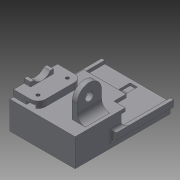
# Autodesk Inventor part: MotorHolder
Saved by Autodesk Inventor 2013 (Build 170138000, 138)
## iProperties
Created: 2013-11-09
Part Number: MotorHolder
Material: Generic
Document SubType Name: Modeling
Designer: JustinIndra
Density: 1 g/cm^3
Author: JustinIndra
Autodesk Inventor part; units mm, degrees
ref_plane "YZ Plane" through (0, 0, 0) normal (1, 0, 0) x (0, 1, 0)
ref_plane "XZ Plane" through (0, 0, 0) normal (0, 1, 0) x (-1, 0, 0)
ref_plane "XY Plane" through (0, 0, 0) normal (0, 0, 1) x (1, 0, 0)
sketch "Sketch1" plane through (0, 0, 0) normal (0, 1, 0) x (-1, 0, 0)
  line L0 (20, 0) -> (-20, 0)
  line L1 (-20, 0) -> (-20, 10)
  line L2 (-20, 10) -> (20, 10)
  line L3 (20, 10) -> (20, 0)
  circle A0 centre (0, 0) radius 3.175
  arc A1 (-20, 0) -> (20, 0) centre (0, 16.3026) ccw
  line L4 (20, 0) -> (-20, 0)
  line L5 (13.2784, -9.5) -> (-17.2645, -9.5) construction
  line L6 (20, 10) -> (-20, 10)
  line L7 (-20, 10) -> (-20, -10)
  line L8 (-20, -10) -> (20, -10)
  line L9 (20, -10) -> (20, 10)
  dimension "d0" = 40
  dimension "d2" = 6.35
  dimension "d4" = 9.5
  dimension "d5" = 10
  dimension "d6" = 20
  constraints: 20 end point, 5 parallel, 3 coincident, 3 perpendicular, 2 centre point, 2 horizontal, 2 point on circle, 1 collinear, 1 midpoint, 1 tangent
  measures "d0" distance of L1.end L2.end
  measures "d2" diameter of A0
  measures "d4" distance between parallel lines of L5 L0
  measures "d5" distance of L0.end L1.end
  measures "d6" distance of L8.end L2.end
extrude "Extrusion1" add sketch "Sketch1" along normal mid plane 8.5 contours L9 L8 L7 A1
sketch "Sketch2" plane through (0, -4.25, 0) normal (0, -1, 0) x (1, 0, 0)
  line L0 (20, -10) -> (20, 0) projected
  line L1 (-20, -10) -> (20, -10)
  line L2 (20, -10) -> (20, 10)
  line L3 (20, 10) -> (-20, 10)
  line L4 (-20, 10) -> (-20, -10)
  point P0 (0, 0)
  dimension "d9" = 20
  constraints: 8 end point, 2 parallel, 1 collinear, 1 horizontal, 1 perpendicular
  measures "d9" distance of L3.end L1.start
extrude "Extrusion2" add sketch "Sketch2" along normal blind 2
sketch "Sketch4" plane through (0, -4.25, 0) normal (0, 1, 0) x (1, 0, 0)
  circle A0 centre (0, 0) radius 3.175
  dimension "d12" = 6.35
  constraints: 1 centre point, 1 coincident
  measures "d12" diameter of A0
extrude "Extrusion3" cut sketch "Sketch4" against normal through all
mirror "Mirror1" about plane through (0, 0, 0) normal (0, 1, 0) of "Extrusion2", "Extrusion3"
sketch "Sketch5" plane through (0, -6.25, 0) normal (0, -1, 0) x (1, 0, 0)
  line L0 (-20, -10) -> (20, -10) projected
  line L1 (-20, 10) -> (-13, 10)
  line L2 (-13, 10) -> (-13, 2.5)
  line L3 (-13, 2.5) -> (-20, 2.5)
  line L4 (-20, 2.5) -> (-20, 10)
  dimension "d15" = 7
  dimension "d17" = 12.5
  constraints: 8 end point, 2 parallel, 1 horizontal, 1 perpendicular
  measures "d15" distance of L2.end L3.end
  measures "d17" distance between parallel lines of L3 L0
extrude "Extrusion4" cut sketch "Sketch5" against normal up to next
mirror "Mirror2" about plane through (0, 0, 0) normal (1, 0, 0) of "Extrusion4"
sketch "Sketch6" plane through (20, -6.25, -10) normal (0, 0, -1) x (-1, 0, 0)
  line L0 (40, 0) -> (40, 12.5) projected
  line L1 (0, 0) -> (40, 0)
  line L2 (40, 0) -> (40, 12.5)
  line L3 (40, 12.5) -> (0, 12.5)
  line L4 (0, 12.5) -> (0, 0)
  point P0 (20, 6.25)
  dimension "d20" = 12.5
  constraints: 8 end point, 2 parallel, 1 horizontal, 1 perpendicular, 1 point on line
  measures "d20" distance of L3.end L1.start
extrude "Extrusion5" add sketch "Sketch6" along normal blind 18.25
sketch "Sketch7" plane through (0, -6.25, 0) normal (0, -1, 0) x (1, 0, 0)
  circle A0 centre (0, 0) radius 3.175 projected
  line L0 (-7.5, -5) -> (-4.5, -5)
  line L1 (-4.5, -5) -> (-4.5, -20)
  line L2 (-4.5, -20) -> (-7.5, -20)
  line L3 (-7.5, -20) -> (-7.5, -5)
  line L4 (10, -5) -> (13, -5)
  line L5 (13, -5) -> (13, -20)
  line L6 (13, -20) -> (10, -20)
  line L7 (10, -20) -> (10, -5)
  dimension "d23" = 15
  dimension "d25" = 3
  dimension "d26" = 4.5
  dimension "d27" = 5
  dimension "d28" = 14.5
  constraints: 16 end point, 4 parallel, 2 equal length, 2 horizontal, 2 perpendicular, 1 collinear
  measures "d23" distance of L2.end L0.start
  measures "d25" distance of L1.end L2.end
  measures "d26" distance from line of A0.centre L1
  measures "d27" distance from line of A0.centre L0
  measures "d28" distance between parallel lines of L1 L7
extrude "Extrusion6" add sketch "Sketch7" along normal blind 17.5 contours L4 L5 L6 L7
sketch "Sketch8" plane through (10, -6.25, -20) normal (-1, 0, 0) x (0, 0, 1)
  line L0 (15, -17.5) -> (0, -17.5)
  circle A0 centre (7.5, -10) radius 2.55
  line L1 (0, 0) -> (15, 0) projected
  line L2 (0, 0) -> (0, -17.5) projected
  line L3 (15, -17.5) -> (0, -17.5) projected
  line L4 (15, 0) -> (15, -17.5) projected
  point P0 (20, 6.25)
  point P1 (7.5, -17.5)
  dimension "d31" = 5.1
  dimension "d34" = 7.5
  constraints: 2 end point, 1 centre point, 1 midpoint, 1 vertical alignment
  measures "d31" diameter of A0
  measures "d34" distance from line of L0 A0.centre
extrude "Extrusion7" cut sketch "Sketch8" against normal through all contours A0
fillet "Fillet1" radius 7.5 2 edges at (11.5, -23.75, -5) (11.5, -23.75, -20)
sketch "Sketch9" plane through (0, -6.25, 0) normal (0, -1, 0) x (1, 0, 0)
  line L0 (10, -20) -> (10, -5) projected
  line L1 (-20, 1) -> (-5, 1)
  line L2 (-5, 1) -> (-5, -26)
  line L3 (-5, -26) -> (-20, -26)
  line L4 (-20, -26) -> (-20, 1)
  line L5 (-20, 2.5) -> (-20, -28.25) projected
  point P0 (-5, -12.5)
  point P1 (10, -12.5)
  dimension "d38" = 15
  dimension "d39" = 27
  constraints: 8 end point, 2 midpoint, 2 parallel, 1 collinear, 1 horizontal, 1 horizontal alignment, 1 perpendicular
  measures "d38" distance between parallel lines of L0 L2
  measures "d39" distance of L3.end L1.start
extrude "Extrusion8" add sketch "Sketch9" along normal blind 4
ref_plane "Work Plane1" through (0, -8.25, 0) normal (0, -1, 0) x (1, 0, 0)
sketch "Sketch10" plane through (0, -8.25, 0) normal (0, -1, 0) x (1, 0, 0)
  line L0 (-7, -4.9434) -> (-9.5, -6.3868)
  line L1 (-9.5, -6.3868) -> (-12, -4.9434)
  line L2 (-12, -4.9434) -> (-12, -2.0566)
  line L3 (-12, -2.0566) -> (-9.5, -0.6132)
  line L4 (-9.5, -0.6132) -> (-7, -2.0566)
  line L5 (-7, -2.0566) -> (-7, -4.9434)
  line L6 (-5, -26) -> (-5, 1) projected
  line L7 (-5, -12.5) -> (-18.5359, -12.5) construction
  line L8 (-12, -3.5) -> (-7, -3.5)
  line L9 (-7, -3.5) -> (-7, 1)
  line L10 (-7, 1) -> (-12, 1)
  line L11 (-12, 1) -> (-12, -3.5)
  line L12 (-5, 1) -> (-20, 1) projected
  point P0 (0, 0)
  point P1 (-9.5, -3.5)
  dimension "d44" = 5
  dimension "d45" = 4.5
  dimension "d46" = 9
  constraints: 22 end point, 2 collinear, 2 midpoint, 2 parallel, 2 perpendicular, 1 horizontal, 1 vertical, 13 other
  measures "d44" distance between parallel lines of L5 L2
  measures "d45" distance from line of L6 point (-9.5, -3.5)
  measures "d46" distance from line of L7 point (-9.5, -3.5)
extrude "Extrusion9" cut sketch "Sketch10" against normal blind 2
ref_plane "Work Plane2" through (-20, -10.25, -12.5) normal (0, 0, 1) x (1, 0, 0)
mirror "Mirror3" about plane through (-20, -10.25, -12.5) normal (0, 0, 1) of "Extrusion9"
sketch "Sketch11" plane through (0, -10.25, 0) normal (0, -1, 0) x (1, 0, 0)
  line L0 (-20, 1) -> (-20, -26) projected
  line L1 (-5, -26) -> (-5, 1) projected
  line L2 (-5, -12.5) -> (-20, -12.5) construction
  point P0 (0, 0)
  point P1 (-9.5, -3.5)
  point P2 (-9.5, -21.5)
  dimension "d49" = 4.5
  dimension "d50" = 18
  constraints: 2 end point, 2 midpoint, 1 symmetric about line
  measures "d49" distance from line of L1 point (-9.5, -3.5)
  measures "d50" distance of point (-9.5, -21.5) point (-9.5, -3.5)
hole "Hole1" at (-9.5, -10.25, -3.5) at (-9.5, -10.25, -21.5) direction (0, 1, 0) diameter 2.013 depth 4 tip angle 118 thread size "M2.5x0.45" class "6H" standard "ISO Metric profile"
sketch "Sketch12" plane through (-20, -4.25, 0) normal (-1, 0, 0) x (0, 0, 1)
  line L0 (-7.5, -6) -> (-17.5, -6)
  line L1 (-17.5, -6) -> (-17.5, -12)
  line L2 (-17.5, -12) -> (-7.5, -12)
  line L3 (-7.5, -12) -> (-7.5, -6)
  line L4 (1, -6) -> (-26, -6) projected
  point P0 (-26, -6.25)
  point P1 (-12.5, -12)
  point P2 (-12.5, -6)
  dimension "d58" = 6
  dimension "d61" = 10
  constraints: 8 end point, 2 midpoint, 2 parallel, 1 collinear, 1 horizontal, 1 perpendicular, 1 vertical alignment
  measures "d58" distance of L0.end L1.end
  measures "d61" distance of L1.end L2.end
extrude "Extrusion10" add sketch "Sketch12" against normal blind 4
sketch "Sketch13" plane through (-20, -6.25, -26) normal (-1, 0, 0) x (0, 0, -1)
  line L0 (-8.5, 10) -> (-18.5, 10) projected
  circle A0 centre (-13.5, 10) radius 6
  point P0 (-26, -6.25)
  dimension "d64" = 12
  constraints: 1 centre point, 1 midpoint
  measures "d64" diameter of A0
extrude "Extrusion11" cut sketch "Sketch13" against normal blind 5
sketch "Sketch14" plane through (-20, -10.25, -7.5) normal (0, 0, 1) x (1, 0, 0)
  line L0 (0, -2.6834) -> (4, -2.6834) projected
  line L1 (4, 0) -> (4, -2.6834) projected
  line L2 (0, 0) -> (4, 0) projected
  line L3 (0, -2.6834) -> (0, 0) projected
  point P0 (20, 10.25)
extrude "Extrusion12" add sketch "Sketch14" along normal blind 2
mirror "Mirror4" about plane through (-20, -10.25, -12.5) normal (0, 0, 1) of "Extrusion12"
fillet "Fillet2" radius 4.5 2 edges at (-5, -8.25, 1) (-5, -8.25, -26)
fillet "Fillet3" radius 5 1 edges at (13, -6.25, -12.5)
fillet "Fillet4" [suppressed]
sketch "Sketch15" plane through (-20, 6.25, 10) normal (0, 0, 1) x (1, 0, 0)
  line L0 (40, 0) -> (0, 0) projected
  line L1 (0, -2) -> (0, 0) projected
  line L2 (40, -2) -> (0, -2) projected
  line L3 (40, -2) -> (40, 0) projected
  point P0 (20, -6.25)
extrude "Extrusion13" add sketch "Sketch15" along normal blind 20
sketch "Sketch16" plane through (-20, 6.25, -28.25) normal (0, 1, 0) x (1, 0, 0)
  line L0 (1.5, -58.25) -> (38.5, -58.25)
  line L1 (38.5, -58.25) -> (38.5, -1.5)
  line L2 (38.5, -1.5) -> (1.5, -1.5)
  line L3 (1.5, -1.5) -> (1.5, -58.25)
  line L4 (0, -58.25) -> (0, 0)
  line L5 (40, -58.25) -> (0, -58.25)
  line L6 (40, 0) -> (40, -58.25)
  line L7 (0, 0) -> (40, 0)
  line L8 (0, -58.25) -> (40, -58.25)
  line L9 (40, -58.25) -> (40, 0)
  line L10 (40, 0) -> (0, 0)
  line L11 (0, 0) -> (0, -58.25)
  circle A0 centre (20, -28.25) radius 3.175
  circle A1 centre (20, -28.25) radius 3.175 projected
  line L12 (0, -58.25) -> (0, 0) projected
  line L13 (40, -58.25) -> (0, -58.25) projected
  line L14 (40, 0) -> (40, -58.25) projected
  line L15 (0, 0) -> (40, 0) projected
  point P0 (20, -1.5)
  point P1 (20, 0)
  dimension "d74" = 37
  dimension "d76" = 56.75
  dimension "d78" = 40
  dimension "d79" = 1.5
  constraints: 24 end point, 4 parallel, 2 collinear, 2 horizontal, 2 midpoint, 2 perpendicular, 2 vertical alignment, 1 centre point
  measures "d74" distance of L0.start L0.end
  measures "d76" distance of L0.end L1.end
  measures "d78" distance of L8.start L8.end
  measures "d79" distance between parallel lines of L2 L10
extrude "Extrusion14" add sketch "Sketch16" along normal blind 4.5 contours L5 L4 L7 L6 L1 L2 L3 | A0
extrude "Extrusion15" cut sketch "Sketch16" along normal blind 4.5 contours L3 L2 L1 L0 | A0
sketch "Sketch18" plane through (18.5, 6.25, -26.75) normal (-1, 0, 0) x (0, 0, 1)
  line L0 (-0.75, 4.25) -> (4.75, 4.25)
  line L1 (4.75, 4.25) -> (4.75, 2.25)
  line L2 (4.75, 2.25) -> (-0.75, 2.25)
  line L3 (-0.75, 2.25) -> (-0.75, 4.25)
  line L4 (23.75, 4.25) -> (29.25, 4.25)
  line L5 (29.25, 4.25) -> (29.25, 2.25)
  line L6 (29.25, 2.25) -> (23.75, 2.25)
  line L7 (23.75, 2.25) -> (23.75, 4.25)
  line L8 (56.75, 0) -> (0, 0) projected
  line L9 (56.75, 4.5) -> (56.75, 0) projected
  line L10 (0, 4.5) -> (56.75, 4.5) projected
  line L11 (0, 0) -> (0, 4.5) projected
  point P0 (26, -6.25)
  dimension "d90" = 2
  dimension "d93" = 5.5
  dimension "d94" = 24.5
  constraints: 16 end point, 4 parallel, 3 collinear, 2 horizontal, 2 perpendicular
  measures "d90" distance of L0.end L1.end
  measures "d93" distance of L0.start L0.end
  measures "d94" distance between parallel lines of L7 L3
extrude "Extrusion17" add sketch "Sketch18" along normal blind 2.25 contours L0 L11 L2 L3 | L0 L1 L2 L11 | L4 L5 L6 L7
sketch "Sketch17" plane through (-20, 6.25, -28.25) normal (0, 1, 0) x (1, 0, 0)
  line L0 (38.5, -58.25) -> (38.5, -1.5) projected
  line L1 (38.5, -35.5) -> (38.25, -35.5)
  line L2 (38.25, -35.5) -> (38.25, -41.5)
  line L3 (38.25, -41.5) -> (38.5, -41.5)
  line L4 (38.5, -41.5) -> (38.5, -35.5)
  line L5 (38.5, -9.5) -> (38.25, -9.5)
  line L6 (38.25, -9.5) -> (38.25, -15.5)
  line L7 (38.25, -15.5) -> (38.5, -15.5)
  line L8 (38.5, -15.5) -> (38.5, -9.5)
  line L9 (1.5, -1.5) -> (38.5, -1.5) projected
  point P0 (38.5, 0)
  dimension "d84" = 8
  dimension "d85" = 6
  dimension "d86" = 20
  dimension "d87" = 0.25
  constraints: 16 end point, 4 parallel, 2 equal length, 2 horizontal, 2 perpendicular, 2 point on line
  measures "d84" distance between parallel lines of L9 L5
  measures "d85" distance of L5.end L6.end
  measures "d86" distance between parallel lines of L7 L1
  measures "d87" distance of L2.end L3.end
extrude "Extrusion16" add sketch "Sketch17" along normal blind 2.5
chamfer "Chamfer1" distance 1 angle 45 2 edges at (16.25, 10.5, -24.375) (16.25, 10.5, -0.25)
mirror "Mirror5" about plane through (0, 0, 0) normal (1, 0, 0) of "Extrusion17", "Extrusion16", "Chamfer1"
sketch "Sketch19" plane through (-20, 6.25, -28.25) normal (0, 1, 0) x (1, 0, 0)
  line L0 (38.5, -58.25) -> (1.5, -58.25) projected
  line L1 (18.25, -49) -> (21.75, -49)
  line L2 (21.75, -49) -> (21.75, -55.5)
  line L3 (21.75, -55.5) -> (18.25, -55.5)
  line L4 (18.25, -55.5) -> (18.25, -49)
  line L5 (17.75, -49) -> (22.25, -49)
  line L6 (22.25, -49) -> (22.25, -56)
  line L7 (22.25, -56) -> (17.75, -56)
  line L8 (17.75, -56) -> (17.75, -49)
  line L9 (1.5, -1.5) -> (38.5, -1.5) projected
  point P0 (20, -56)
  point P1 (20, -55.5)
  point P2 (20, -58.25)
  point P3 (40, -58.25)
  point P4 (0, -58.25)
  dimension "d100" = 54.5
  dimension "d101" = 0.5
  dimension "d102" = 0.5
  dimension "d103" = 7
  dimension "d104" = 3.5
  constraints: 16 end point, 4 parallel, 3 midpoint, 2 horizontal, 2 perpendicular, 2 vertical alignment, 1 collinear
  measures "d100" distance between parallel lines of L9 L7
  measures "d101" distance between parallel lines of L7 L3
  measures "d102" distance between parallel lines of L6 L2
  measures "d103" distance of L7.end L5.start
  measures "d104" distance of L2.end L3.end
extrude "Extrusion18" cut sketch "Sketch19" against normal through all contours L4 L3 L2 L5 L6 L7 L8
sketch "Sketch20" plane through (0, 4.25, 16.3026) normal (0, -1, 0) x (1, 0, 0)
  line L0 (-1.75, 10.9474) -> (1.75, 10.9474)
  line L1 (1.75, 10.9474) -> (1.75, 4.4474)
  line L2 (1.75, 4.4474) -> (-1.75, 4.4474)
  line L3 (-1.75, 4.4474) -> (-1.75, 10.9474)
  constraints: 8 end point, 2 parallel, 1 horizontal, 1 perpendicular
extrude "Extrusion19" cut sketch "Sketch20" against normal blind 1
fillet "Fillet5" radius 2 1 edges at (0, 5.25, 20.75)
sketch "Sketch21" plane through (-1.75, 6.25, 20.75) normal (-1, 0, 0) x (0, 0, 1)
  line L0 (0, 0) -> (6.5, 0) projected
  line L1 (6.5, 0) -> (4, 0)
  line L2 (4, 1) -> (4, 0)
  line L3 (4, 1) -> (6.5, 0)
  point P0 (-20.75, -6.25)
  dimension "d110" = 1
  dimension "d111" = 2.5
  constraints: 6 end point, 1 perpendicular, 1 point on line
  measures "d110" distance of L2.start L1.end
  measures "d111" distance of L0.end L1.end
extrude "Extrusion20" add sketch "Sketch21" against normal up to surface (3.5 mm away)
sketch "Sketch23" plane through (-18.5, 6.25, 30) normal (0, 1, 0) x (1, 0, 0)
  line L0 (37, 48.75) -> (37, 56.75) projected
  line L1 (37, 56.75) -> (0, 56.75) projected
  line L2 (18, 56.75) -> (18.5, 56.75)
  line L3 (18.5, 56.75) -> (18.5, 52.5)
  line L4 (18.5, 52.5) -> (18, 52.5)
  line L5 (18, 52.5) -> (18, 56.75)
  line L6 (20.25, 56.75) -> (20.75, 56.75)
  line L7 (20.75, 56.75) -> (20.75, 52.5)
  line L8 (20.75, 52.5) -> (20.25, 52.5)
  line L9 (20.25, 52.5) -> (20.25, 56.75)
  dimension "d114" = 16.25
  dimension "d116" = 18.5
  dimension "d117" = 1.75
  dimension "d118" = 4.25
  constraints: 16 end point, 4 parallel, 2 equal length, 2 horizontal, 2 perpendicular, 2 point on line
  measures "d114" distance between parallel lines of L0 L7
  measures "d116" distance between parallel lines of L0 L3
  measures "d117" distance between parallel lines of L9 L3
  measures "d118" distance of L4.end L2.start
extrude "Extrusion21" cut sketch "Sketch23" against normal blind 5
sketch "Sketch24" plane through (0, 4.25, 16.3026) normal (0, -1, 0) x (1, 0, 0)
  line L0 (-20, 13.6974) -> (-22, 13.6974)
  line L1 (-22, 13.6974) -> (-22, -21.3026)
  line L2 (-22, -21.3026) -> (-20, -21.3026)
  line L3 (-20, -21.3026) -> (-20, 13.6974)
  dimension "d121" = 2
  dimension "d122" = 35
  constraints: 8 end point, 2 parallel, 1 horizontal, 1 perpendicular
  measures "d121" distance of L0.start L0.end
  measures "d122" distance of L0.end L1.end
extrude "Extrusion22" add sketch "Sketch24" along normal mid plane 4
mirror "Mirror6" about plane through (0, 0, 0) normal (1, 0, 0) of "Extrusion22"
fillet "Fillet6" radius 2 6 edges at (-20, 4.25, -5) (-20, 6.25, 12.5) (-20, 2.25, -2.5) (20, 4.25, -5) (20, 6.25, 12.5) (20, 2.25, -2.5)
equation "\"d6\" = 2 * d5"
equation "\"d78\" = d74 + 2 * d79"
equation "\"d102\" = d101"
body "Solid1"
